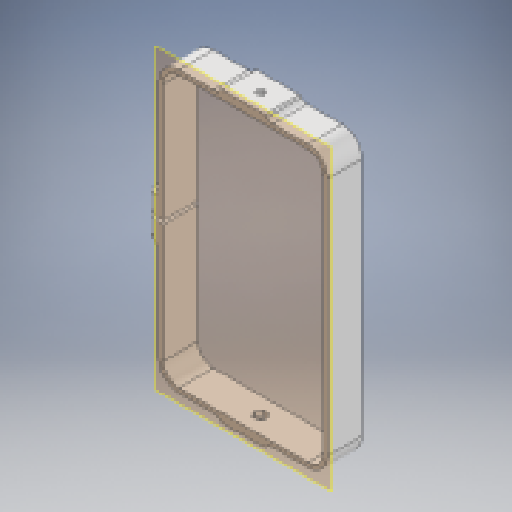
# Autodesk Inventor part: Fascia
Saved by Autodesk Inventor 2024 (Build 280153000, 153)
## iProperties
Created: 2024-08-21
Part Number: Fascia
Material: Generic
Document SubType Name: Modeling
Designer: Stefano
Density: 1 g/cm^3
Appearance: Default
Author: Stefano
Autodesk Inventor part; units mm, degrees
ref_plane "YZ Plane" through (0, 0, 0) normal (1, 0, 0) x (0, 1, 0)
ref_plane "XZ Plane" through (0, 0, 0) normal (0, 1, 0) x (-1, 0, 0)
ref_plane "XY Plane" through (0, 0, 0) normal (0, 0, 1) x (1, 0, 0)
ref_plane "Work Plane1" through (0, 0, 0) normal (0, 0, 1) x (1, 0, 0)
sketch "Sketch1" plane through (0, 0, 0) normal (0, 0, 1) x (1, 0, 0)
  line L0 (-47.5, 96.9) -> (47.5, 96.9) projected
  arc A0 (55.9, 88.5) -> (47.5, 96.9) centre (47.5, 88.5) ccw projected
  line L1 (55.9, 88.5) -> (55.9, -88.5) projected
  arc A1 (47.5, -96.9) -> (55.9, -88.5) centre (47.5, -88.5) ccw projected
  line L2 (47.5, -96.9) -> (-47.5, -96.9) projected
  arc A2 (-55.9, -88.5) -> (-47.5, -96.9) centre (-47.5, -88.5) ccw projected
  line L3 (-55.9, -88.5) -> (-55.9, 88.5) projected
  arc A3 (-47.5, 96.9) -> (-55.9, 88.5) centre (-47.5, 88.5) ccw projected
  arc A4 (58.9, 88.5) -> (47.5, 99.9) centre (47.5, 88.5) ccw projected
  line L4 (47.5, 99.9) -> (-47.5, 99.9) projected
  arc A5 (-47.5, 99.9) -> (-58.9, 88.5) centre (-47.5, 88.5) ccw projected
  line L5 (-58.9, 88.5) -> (-58.9, -88.5) projected
  arc A6 (-58.9, -88.5) -> (-47.5, -99.9) centre (-47.5, -88.5) ccw projected
  line L6 (-47.5, -99.9) -> (47.5, -99.9) projected
  arc A7 (47.5, -99.9) -> (58.9, -88.5) centre (47.5, -88.5) ccw projected
  line L7 (58.9, -88.5) -> (58.9, 88.5) projected
  line L8 (-47.5, 103.075) -> (47.5, 103.075)
  arc A8 (62.075, 88.5) -> (47.5, 103.075) centre (47.5, 88.5) ccw
  line L9 (62.075, 88.5) -> (62.075, -88.5)
  arc A9 (47.5, -103.075) -> (62.075, -88.5) centre (47.5, -88.5) ccw
  line L10 (47.5, -103.075) -> (-47.5, -103.075)
  arc A10 (-62.075, -88.5) -> (-47.5, -103.075) centre (-47.5, -88.5) ccw
  line L11 (-62.075, -88.5) -> (-62.075, 88.5)
  arc A11 (-47.5, 103.075) -> (-62.075, 88.5) centre (-47.5, 88.5) ccw
  line L12 (0, 103.075) -> (0, -103.075) construction
  line L13 (19.05, 103.075) -> (15.875, 106.25)
  line L14 (15.875, 106.25) -> (-15.875, 106.25)
  line L15 (-15.875, 106.25) -> (-19.05, 103.075)
  line L16 (62.075, 0) -> (-62.075, 0) construction
  line L17 (19.05, -103.075) -> (15.875, -106.25)
  line L18 (15.875, -106.25) -> (-15.875, -106.25)
  line L19 (-15.875, -106.25) -> (-19.05, -103.075)
  line L20 (-62.075, 1.27) -> (-71.6, 1.27)
  line L21 (-71.6, 1.27) -> (-71.6, 13.97)
  line L22 (-71.6, 13.97) -> (-62.075, 13.97)
  line L23 (-55.9, 88.5) -> (-55.9, -88.5)
  line L24 (-62.075, -1.27) -> (-71.6, -1.27)
  line L25 (-71.6, -1.27) -> (-71.6, -13.97)
  line L26 (-71.6, -13.97) -> (-62.075, -13.97)
  line L27 (-62.075, 1.27) -> (-58.9, 1.27)
  line L28 (-62.075, -1.27) -> (-58.9, -1.27)
  point P0 (0, 0)
  dimension "d0" = 3.175
  dimension "d1" = 38.1
  dimension "d2" = 3.175
  dimension "d3" = 45
  dimension "d4" = 9.525
  dimension "d5" = 1.27
  dimension "d6" = 12.7
  constraints: 42 end point, 10 symmetric about line, 8 point on circle, 6 point on line, 5 perpendicular, 4 centre point, 4 midpoint, 1 horizontal, 8 other
  measures "d0" distance between parallel lines of L4 L8
  measures "d1" distance of L15.end L13.start
  measures "d2" distance from line of L8 L13.end
  measures "d3" angle of L8 L15
  measures "d4" distance between parallel lines of L11 L21
  measures "d5" distance between parallel lines of L20 L16
  measures "d6" distance between parallel lines of L22 L20
extrude "Extrusion1" add sketch "Sketch1" against normal blind 25.4 contours A4 L4 A5 L5 L27 L11 A11 L8 A8 L9 A9 L10 A10 L28 A6 L6 A7 L7 | L20 L21 L22 L11 | L11 L26 L25 L24 | L15 L14 L13 L8 | L10 L17 L18 L19
sketch "Sketch2" plane through (-71.6, 13.97, 0) normal (0, 1, 0) x (1, 0, 0)
  line L0 (0, 0) -> (9.525, 0) construction
  line L1 (4.7625, 0) -> (4.7625, 25.4) construction
  line L2 (9.525, 25.4) -> (0, 25.4) construction
  point P0 (71.6, 0)
  point P1 (4.7625, 12.7)
  constraints: 3 midpoint, 2 end point
hole "Hole1" at (-66.8375, 13.97, -12.7) direction (0, -1, 0) diameter 3.6068 depth 12.7 tip angle 118 counterbore diameter 6.5024 counterbore depth 2.9972 clearance for "Socket Head Cap Screw" size "M3" standard "Ansi Metric M Profile"
sketch "Sketch6" plane through (-71.6, -13.97, 0) normal (0, -1, 0) x (1, 0, 0)
  line L0 (4.7625, -15.9332) -> (1.9625, -14.3166)
  line L1 (1.9625, -14.3166) -> (1.9625, -11.0834)
  line L2 (1.9625, -11.0834) -> (4.7625, -9.4668)
  line L3 (4.7625, -9.4668) -> (7.5625, -11.0834)
  line L4 (7.5625, -11.0834) -> (7.5625, -14.3166)
  line L5 (7.5625, -14.3166) -> (4.7625, -15.9332)
  point P0 (71.6, 0)
  point P1 (4.7625, -12.7)
  point P2 (4.7625, -12.7)
  dimension "d39" = 5.6
  constraints: 12 end point, 1 coincident, 13 other
  measures "d39" distance between parallel lines of L4 L1
extrude "Extrusion3" cut sketch "Sketch6" against normal blind 4
sketch "Sketch7" plane through (-71.6, -9.97, 0) normal (0, -1, 0) x (1, 0, 0)
  point P0 (71.6, 0)
  point P1 (4.7625, -12.7)
hole "Hole4" at (-66.8375, -9.97, -12.7) direction (0, 1, 0) diameter 3.4036 depth 8.7 tip angle 118 clearance for "Socket Head Cap Screw" size "M3" standard "Ansi Metric M Profile"
fillet "Fillet1" radius 6.35 4 edges at (-71.6, 7.62, 0) (-71.6, 7.62, -25.4) (-71.6, -7.62, -25.4) (-71.6, -7.62, 0)
fillet "Fillet2" radius 6.35 6 edges at (-62.075, 13.97, -12.7) (-62.075, -13.97, -12.7) (-19.05, -103.075, -12.7) (19.05, -103.075, -12.7) (19.05, 103.075, -12.7) (-19.05, 103.075, -12.7)
sketch "Sketch3" plane through (-47.5, -99.9, 0) normal (0, 1, 0) x (1, 0, 0)
  line L0 (31.625, 0) -> (63.375, 0) construction
  line L1 (31.625, 0) -> (31.625, 25.4) construction
  line L2 (63.375, 25.4) -> (31.625, 25.4) construction
  line L3 (63.375, 0) -> (63.375, 25.4) construction
  line L4 (63.375, 0) -> (63.375, 25.4) construction
  line L5 (63.375, 12.7) -> (31.625, 12.7) construction
  line L6 (42.8235, 12.7) -> (45.1617, 16.75)
  line L7 (45.1617, 16.75) -> (49.8383, 16.75)
  line L8 (49.8383, 16.75) -> (52.1765, 12.7)
  line L9 (52.1765, 12.7) -> (49.8383, 8.65)
  line L10 (49.8383, 8.65) -> (45.1617, 8.65)
  line L11 (45.1617, 8.65) -> (42.8235, 12.7)
  point P0 (47.5, 0)
  point P1 (47.5, 12.7)
  point P2 (47.5, 12.7)
  dimension "d18" = 8.1
  constraints: 14 end point, 3 midpoint, 1 coincident, 1 point on line, 13 other
  measures "d18" distance between parallel lines of L10 L7
extrude "Extrusion2" cut sketch "Sketch3" against normal blind 4
sketch "Sketch4" plane through (-47.5, -103.9, 0) normal (0, 1, 0) x (1, 0, 0)
  line L0 (45.1617, 16.75) -> (49.8383, 16.75) construction
  line L1 (45.1617, 8.65) -> (42.8235, 12.7) construction
  line L2 (49.8383, 16.75) -> (45.1617, 8.65) construction
  point P0 (47.5, 0)
  point P1 (47.5, 12.7)
  constraints: 2 end point, 1 midpoint
hole "Hole2" at (0, -103.9, -12.7) direction (0, -1, 0) diameter 5.5118 end through all clearance for "Socket Head Cap Screw" size "M5" standard "Ansi Metric M Profile"
mirror "Mirror1" about plane through (0, 0, 0) normal (0, 1, 0) of "Extrusion2", "Hole2"
body "Solid1"
